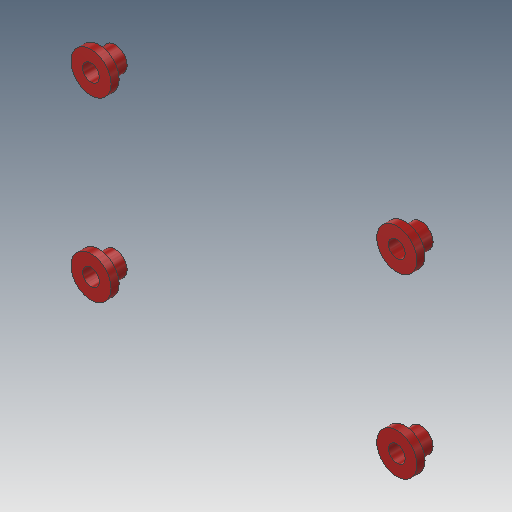
# Autodesk Inventor part: battery_lib_hook
Saved by Autodesk Inventor 2019.4 (Build 234330000, 330)
## iProperties
Created: 2019-01-22
Part Number: battery_lib_hook
Material: 一般
Document SubType Name: Modeling
Designer: y6tada
Density: 1 g/cm^3
Appearance: 赤
Mass: 0.0935252 g
Surface Area: 3.46769 cm^2
Volume: 0.0935252 cm^3
Author: y6tada
Autodesk Inventor part; units mm, degrees
ref_plane "YZ Plane" through (0, 0, 0) normal (1, 0, 0) x (0, 1, 0)
ref_plane "XZ Plane" through (0, 0, 0) normal (0, 1, 0) x (-1, 0, 0)
ref_plane "XY Plane" through (0, 0, 0) normal (0, 0, 1) x (1, 0, 0)
sketch "スケッチ1" plane through (0, 0, 0) normal (0, 0, 1) x (1, 0, 0)
  circle A0 centre (-19, 9) radius 1.05
  circle A1 centre (19, 9) radius 1.05
  circle A2 centre (-19, -13) radius 1.05
  circle A3 centre (19, -13) radius 1.05
  circle A4 centre (-19, 9) radius 1.5
  circle A5 centre (-19, -13) radius 1.5
  circle A6 centre (19, -13) radius 1.5
  circle A7 centre (19, 9) radius 1.5
  circle A8 centre (-19, 9) radius 0.8 construction
  circle A9 centre (-19, -13) radius 0.8 construction
  line L0 (0, 0) -> (0, 11.6821) construction
  dimension "d0" = 2.1
  dimension "d3" = 3
  constraints: 8 centre point, 6 equal radius, 4 coincident, 2 concentric, 2 end point, 2 symmetric about line, 1 vertical
  measures "d0" diameter of A0
  measures "d3" diameter of A4
extrude "押し出し1" add sketch "スケッチ1" along normal blind 2
sketch "スケッチ2" plane through (-19, 9, 2) normal (0, 0, 1) x (1, 0, 0)
  circle A0 centre (0, 0) radius 1.05 projected
  circle A1 centre (0, -22) radius 1.05 projected
  circle A2 centre (38, -22) radius 1.05 projected
  circle A3 centre (38, 0) radius 1.05 projected
  circle A4 centre (0, 0) radius 1.05 projected
  circle A5 centre (0, 0) radius 2.5
  circle A6 centre (0, -22) radius 2.5
  circle A7 centre (38, -22) radius 2.5
  circle A8 centre (38, 0) radius 2.5
  point P0 (19, -9)
  dimension "d4" = 5
  constraints: 4 centre point, 4 coincident, 3 equal radius
  measures "d4" diameter of A5
extrude "押し出し2" add sketch "スケッチ2" along normal blind 1
